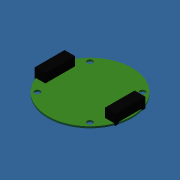
# Autodesk Inventor part: Encoder without LEDs
Saved by Autodesk Inventor 2016 (Build 200138000, 138)
## iProperties
Company: betabots
Created: 2015-01-07
Part Number: Encoder without LEDs
Material: Generisch
Document SubType Name: Modeling
Designer: 4ndreas
Density: 1 g/cm^3
Appearance: PCB- green
Mass: 3.05798 g
Surface Area: 48.0346 cm^2
Volume: 3.05798 cm^3
Description: Encoder without LEDs
Author: 4ndreas
Title: Encoder PCB
Autodesk Inventor part; units mm, degrees
ref_plane "YZ Plane" through (0, 0, 0) normal (1, 0, 0) x (0, 1, 0)
ref_plane "XZ Plane" through (0, 0, 0) normal (0, 1, 0) x (-1, 0, 0)
ref_plane "XY Plane" through (0, 0, 0) normal (0, 0, 1) x (1, 0, 0)
sketch "Skizze1" plane through (0, 0, 0) normal (0, 0, 1) x (1, 0, 0)
  circle A0 centre (0, 0) radius 25
  circle A1 centre (0, 0) radius 23.984
  circle A2 centre (0, 0) radius 21.2132 construction
  line L0 (-15, 15) -> (15, 15) construction
  line L1 (15, 15) -> (15, -15) construction
  line L2 (15, -15) -> (-15, -15) construction
  line L3 (-15, -15) -> (-15, 15) construction
  point P0 (15, 15)
  point P1 (15, -15)
  dimension "d0" = 50
  dimension "d1" = 1.016
  dimension "d2" = 30
  constraints: 8 end point, 6 coincident, 4 point on circle, 3 centre point, 2 parallel, 2 perpendicular, 1 horizontal, 1 point on line
  measures "d0" diameter of A0
  measures "d1" radial gap between concentric circles of A0 A1
  measures "d2" distance between parallel lines of L1 L3
extrude "Extrusion1" add sketch "Skizze1" against normal blind 1 contours A1
hole "Bohrung1" at (-15, 15, 0) at (15, 15, 0) at (15, -15, 0) at (-15, -15, 0) direction (0, 0, -1) diameter 3.2 end through all
sketch "Skizze2" plane through (0, 0, 0) normal (0, 0, 1) x (1, 0, 0)
  circle A0 centre (15, -15) radius 1.6 projected
  circle A1 centre (-15, 15) radius 1.6 projected
  circle A2 centre (15, 15) radius 1.6 projected
  circle A3 centre (-15, -15) radius 1.6 projected
  circle A4 centre (0, 0) radius 23.984 projected
  line L0 (-25.6213, 25.3721) -> (25.184, 25.3721) construction
  line L1 (25.184, 25.3721) -> (25.184, -25.4332) construction
  line L2 (25.184, -25.4332) -> (-25.6213, -25.4332) construction
  line L3 (-25.6213, -25.4332) -> (-25.6213, 25.3721) construction
  constraints: 1 horizontal, 2 other
sketch "Skizze3" plane through (0, 0, 0) normal (0, 0, 1) x (1, 0, 0)
  circle A0 centre (0, 0) radius 23.984 projected
  line L0 (-2.5, 2.5) -> (2.5, 2.5)
  line L1 (2.5, 2.5) -> (2.5, -2.5)
  line L2 (2.5, -2.5) -> (-2.5, -2.5)
  line L3 (-2.5, -2.5) -> (-2.5, 2.5)
  line L4 (-15, 2.5) -> (-10, 2.5)
  line L5 (-10, 2.5) -> (-10, -2.5)
  line L6 (-10, -2.5) -> (-15, -2.5)
  line L7 (-15, -2.5) -> (-15, 2.5)
  line L8 (-15, 2.5) -> (-10, -2.5) construction
  line L9 (-2.5, 2.5) -> (2.5, -2.5) construction
  line L10 (2.5, -2.5) -> (0, 0) construction
  line L11 (0, 0) -> (-12.5, 0) construction
  line L12 (-2.5, -15) -> (-2.5, -10)
  line L13 (-2.5, -10) -> (2.5, -10)
  line L14 (2.5, -10) -> (2.5, -15)
  line L15 (2.5, -15) -> (-2.5, -15)
  line L16 (15, -2.5) -> (10, -2.5)
  line L17 (10, -2.5) -> (10, 2.5)
  line L18 (10, 2.5) -> (15, 2.5)
  line L19 (15, 2.5) -> (15, -2.5)
  line L20 (2.5, 15) -> (2.5, 10)
  line L21 (2.5, 10) -> (-2.5, 10)
  line L22 (-2.5, 10) -> (-2.5, 15)
  line L23 (-2.5, 15) -> (2.5, 15)
  dimension "d24" = 5
  dimension "d25" = 12.5
  dimension "d28" = 360
  constraints: 49 end point, 5 parallel, 3 equal length, 3 horizontal, 2 midpoint, 2 perpendicular, 1 collinear, 33 other
  measures "d24" distance between parallel lines of L1 L3
  measures "d25" distance of L10.end L11.end
extrude "Extrusion2" [suppressed]
sketch "Skizze4" plane through (0, 0, -1) normal (0, 0, -1) x (-1, 0, 0)
  circle A0 centre (0, 0) radius 23.984 projected
  line L0 (-2.95, 2.5) -> (2.95, 2.5)
  line L1 (2.95, 2.5) -> (2.95, -2.5)
  line L2 (2.95, -2.5) -> (-2.95, -2.5)
  line L3 (-2.95, -2.5) -> (-2.95, 2.5)
  line L4 (-2.95, -2.5) -> (2.95, 2.5) construction
  dimension "d33" = 5.9
  dimension "d34" = 5
  constraints: 10 end point, 2 parallel, 1 coincident, 1 horizontal, 1 midpoint, 1 perpendicular
  measures "d33" distance between parallel lines of L3 L1
  measures "d34" distance between parallel lines of L2 L0
extrude "Extrusion3" add sketch "Skizze4" along normal blind 2 separate body contours L0 L1 L2 L3
sketch "Skizze5" plane through (0, 0, -1) normal (0, 0, -1) x (-1, 0, 0)
  circle A0 centre (0, 0) radius 23.984 projected
  line L0 (-23, 8.5) -> (-17, 8.5)
  line L1 (-17, 8.5) -> (-17, -8.5)
  line L2 (-17, -8.5) -> (-23, -8.5)
  line L3 (-23, -8.5) -> (-23, 8.5)
  line L4 (17, 8.5) -> (23, 8.5)
  line L5 (23, 8.5) -> (23, -8.5)
  line L6 (23, -8.5) -> (17, -8.5)
  line L7 (17, -8.5) -> (17, 8.5)
  line L8 (-23, 0) -> (23, 0) construction
  line L9 (-20, 8.5) -> (-20, -8.5) construction
  point P0 (0, 0)
  dimension "d38" = 17
  dimension "d39" = 6
  dimension "d40" = 20
  constraints: 20 end point, 5 midpoint, 4 parallel, 3 perpendicular, 2 equal length, 2 horizontal, 1 coincident
  measures "d38" distance between parallel lines of L2 L0
  measures "d39" distance between parallel lines of L3 L1
  measures "d40" distance from line of L9 A0.centre
extrude "Extrusion4" add sketch "Skizze5" against normal blind 6 contours L5 A0 L6 L7 L4 | A0 L4 L5 | L5 L6 A0 | L0 L1 L2 A0 L3 | A0 L3 L0 | L2 L3 A0 bodies 2
sketch "Skizze6" plane through (0, 0, -1) normal (0, 0, -1) x (-1, 0, 0)
  line L0 (-26.2075, 26.1914) -> (26.4628, 26.1914) construction
  line L1 (26.4628, 26.1914) -> (26.4628, -26.479) construction
  line L2 (26.4628, -26.479) -> (-26.2075, -26.479) construction
  line L3 (-26.2075, -26.479) -> (-26.2075, 26.1914) construction
  constraints: 1 horizontal, 2 other
ref_plane "Arbeitsebene1" through (-15, -15, -67.8444) normal (-0.7071, 0.7071, 0) x (0, 0, 1)
